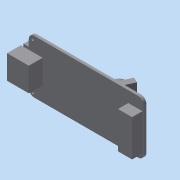
# Autodesk Inventor part: 00_ESP32_CAM
Saved by Autodesk Inventor 2019.4 (Build 234330000, 330)
## iProperties
Created: 2020-11-30
Part Number: 00_ESP32_CAM
Material: Generic
Document SubType Name: Modeling
Designer: diederichbenedict
Density: 1 g/cm^3
Appearance: Default
Author: diederichbenedict
Autodesk Inventor part; units mm, degrees
ref_plane "YZ Plane" through (0, 0, 0) normal (1, 0, 0) x (0, 1, 0)
ref_plane "XZ Plane" through (0, 0, 0) normal (0, 1, 0) x (-1, 0, 0)
ref_plane "XY Plane" through (0, 0, 0) normal (0, 0, 1) x (1, 0, 0)
sketch "Sketch1" plane through (0, 0, 0) normal (0, 0, 1) x (1, 0, 0)
  line L0 (19.65, -10.075) -> (-19.65, -10.075)
  line L1 (-21.65, -8.075) -> (-21.65, 8.075)
  line L2 (-19.65, 10.075) -> (19.65, 10.075)
  line L3 (21.65, 8.075) -> (21.65, -8.075)
  line L4 (21.65, -10.075) -> (-21.65, 10.075) construction
  line L5 (-21.65, -10.075) -> (21.65, 10.075) construction
  arc A0 (-19.65, 10.075) -> (-21.65, 8.075) centre (-19.65, 8.075) ccw
  arc A1 (21.65, 8.075) -> (19.65, 10.075) centre (19.65, 8.075) ccw
  arc A2 (19.65, -10.075) -> (21.65, -8.075) centre (19.65, -8.075) ccw
  arc A3 (-21.65, -8.075) -> (-19.65, -10.075) centre (-19.65, -8.075) ccw
  point P0 (0, 0)
  dimension "d0" = 43.3
  dimension "d1" = 20.15
  dimension "d2" = 2
  constraints: 12 end point, 8 point on circle, 8 point on line, 8 tangent, 4 centre point, 3 equal radius, 2 midpoint, 2 parallel, 1 horizontal, 1 perpendicular
  measures "d0" distance of L4.end L5.end
  measures "d1" distance of L5.start L4.end
  measures "d2" radius of A0
extrude "Extrusion1" add sketch "Sketch1" along normal blind 1
sketch "Sketch2" plane through (0, 0, 0) normal (0, 0, -1) x (-1, 0, 0)
  line L0 (19.65, 10.075) -> (-19.65, 10.075) projected
  arc A0 (-19.65, 10.075) -> (-21.65, 8.075) centre (-19.65, 8.075) ccw projected
  line L1 (-21.65, 8.075) -> (-21.65, -8.075) projected
  arc A1 (-21.65, -8.075) -> (-19.65, -10.075) centre (-19.65, -8.075) ccw projected
  line L2 (-19.65, -10.075) -> (19.65, -10.075) projected
  arc A2 (19.65, -10.075) -> (21.65, -8.075) centre (19.65, -8.075) ccw projected
  line L3 (21.65, -8.075) -> (21.65, 8.075) projected
  arc A3 (21.65, 8.075) -> (19.65, 10.075) centre (19.65, 8.075) ccw projected
  line L4 (17.25, -4.5) -> (24.65, -4.5)
  line L5 (24.65, -4.5) -> (24.65, 4.5)
  line L6 (24.65, 4.5) -> (17.25, 4.5)
  line L7 (17.25, 4.5) -> (17.25, -4.5)
  line L8 (17.25, -4.5) -> (24.65, 4.5) construction
  line L9 (24.65, -4.5) -> (17.25, 4.5) construction
  point P0 (0, 0)
  point P1 (20.95, 0)
  dimension "d5" = 7.4
  dimension "d6" = 9
  dimension "d7" = 3
  constraints: 12 end point, 2 midpoint, 2 parallel, 1 horizontal, 1 perpendicular
  measures "d5" distance of L6.end L5.end
  measures "d6" distance of L5.end L4.end
  measures "d7" distance between parallel lines of L3 L5
extrude "Extrusion2" add sketch "Sketch2" along normal blind 3 contours L6 L5 L4 L3 | L3 L4 L7 L6
sketch "Sketch3" plane through (0, 0, 1) normal (0, 0, 1) x (1, 0, 0)
  line L0 (-16.45, 4.5) -> (-24.65, 4.5)
  line L1 (-24.65, 4.5) -> (-24.65, -4.5)
  line L2 (-24.65, -4.5) -> (-16.45, -4.5)
  line L3 (-16.45, -4.5) -> (-16.45, 4.5)
  line L4 (-16.45, 4.5) -> (-24.65, -4.5) construction
  line L5 (-24.65, 4.5) -> (-16.45, -4.5) construction
  line L6 (-21.65, 8.075) -> (-21.65, -8.075) projected
  point P0 (0, 0)
  point P1 (-20.55, 0)
  dimension "d10" = 8.2
  dimension "d11" = 9
  dimension "d12" = 3
  constraints: 12 end point, 2 midpoint, 2 parallel, 1 horizontal, 1 perpendicular
  measures "d10" distance of L2.end L1.end
  measures "d11" distance of L1.end L0.end
  measures "d12" distance between parallel lines of L6 L1
extrude "Extrusion3" add sketch "Sketch3" along normal blind 5.2
sketch "Sketch4" plane through (0, 0, 1) normal (0, 0, 1) x (1, 0, 0)
  line L0 (21.1704, -7.925) -> (15.85, -7.925)
  line L1 (15.85, -7.925) -> (15.85, 5.875)
  line L2 (15.85, 5.875) -> (21.1704, 5.875)
  line L3 (21.1704, 5.875) -> (21.1704, -7.925)
  line L4 (-19.65, -10.075) -> (19.65, -10.075) projected
  line L5 (19.65, 10.075) -> (-19.65, 10.075) projected
  line L6 (21.65, -8.075) -> (21.65, 8.075) projected
  point P0 (0, 0)
  dimension "d15" = 2.15
  dimension "d16" = 4.2
  dimension "d17" = 5.8
  constraints: 8 end point, 2 parallel, 1 horizontal, 1 perpendicular
  measures "d15" distance between parallel lines of L0 L4
  measures "d16" distance between parallel lines of L2 L5
  measures "d17" distance between parallel lines of L6 L1
extrude "Extrusion4" add sketch "Sketch4" along normal blind 3.9
sketch "Sketch5" plane through (0, 0, 0) normal (0, 0, -1) x (-1, 0, 0)
  line L0 (17.25, 4.5) -> (21.65, 4.5) projected
  line L1 (21.65, 4.5) -> (21.65, 8.075) projected
  arc A0 (21.65, 8.075) -> (19.65, 10.075) centre (19.65, 8.075) ccw projected
  line L2 (19.65, 10.075) -> (-19.65, 10.075) projected
  arc A1 (-19.65, 10.075) -> (-21.65, 8.075) centre (-19.65, 8.075) ccw projected
  line L3 (-21.65, 8.075) -> (-21.65, -8.075) projected
  arc A2 (-21.65, -8.075) -> (-19.65, -10.075) centre (-19.65, -8.075) ccw projected
  line L4 (-19.65, -10.075) -> (19.65, -10.075) projected
  arc A3 (19.65, -10.075) -> (21.65, -8.075) centre (19.65, -8.075) ccw projected
  line L5 (21.65, -8.075) -> (21.65, -4.5) projected
  line L6 (21.65, -4.5) -> (17.25, -4.5) projected
  line L7 (17.25, -4.5) -> (17.25, 4.5) projected
  circle A4 centre (20.3112, 8.6013) radius 0.5
  circle A5 centre (20.3112, -8.8284) radius 0.5
  point P0 (0, 0)
  dimension "d20" = 1
  dimension "d21" = 1
  constraints: 2 centre point
  measures "d20" diameter of A4
  measures "d21" diameter of A5
extrude "Extrusion5" cut sketch "Sketch5" against normal blind 3.9 contours A4 | A5
sketch "Sketch6" plane through (0, 0, 0) normal (0, 1, 0) x (-1, 0, 0)
  line L0 (19.65, 0) -> (-19.65, 0) projected
  line L1 (-3.7519, 0) -> (-2.2949, -8.2628)
  line L2 (21.65, 0) -> (21.65, 1) projected
  line L3 (-3.6651, -0.4924) -> (-2.0849, -9.4542)
  line L4 (-2.0849, -9.4542) -> (0.1802, -9.0548)
  line L5 (0.1802, -9.0548) -> (-1.4, -0.093)
  line L6 (-1.4, -0.093) -> (-3.6651, -0.4924)
  line L7 (-3.6651, -0.4924) -> (0.1802, -9.0548) construction
  line L8 (-2.0849, -9.4542) -> (-1.4, -0.093) construction
  line L9 (-21.65, 0) -> (-21.65, 1) projected
  point P0 (0, 0)
  point P1 (-1.7424, -4.7736)
  dimension "deg_1" = 80
  dimension "d28" = 9.1
  dimension "d29" = 2.3
  dimension "d30" = 0.5
  dimension "d42" = 20.25
  constraints: 14 end point, 2 midpoint, 2 parallel, 2 point on line, 1 collinear, 1 perpendicular
  measures "deg_1" angle of L0 L1
  measures "d28" distance of L3.start L3.end
  measures "d29" distance of L4.end L3.end
  measures "d30" distance from line of L1.start L6
  measures "d42" distance from line of L9 L5.end
extrude "Extrusion6" add sketch "Sketch6" along normal mid plane 9.1
sketch "Sketch7" plane through (1.4, -4.55, -0.093) normal (-0.9848, 0, 0.1736) x (0.1736, 0, 0.9848)
  line L0 (0, 9.1) -> (0, 0) projected
  line L1 (-9.1, 9.1) -> (0, 9.1) projected
  line L2 (-9.1, 9.1) -> (-9.1, 0) projected
  line L3 (0, 0) -> (-9.1, 0) projected
  circle A0 centre (-4.55, 4.55) radius 4.15
  circle A1 centre (-4.55, 4.55) radius 3.5
  point P0 (-0.1515, 4.55)
  dimension "d33" = 8.3
  dimension "d34" = 7
  constraints: 2 centre point, 1 coincident
  measures "d33" diameter of A0
  measures "d34" diameter of A1
extrude "Extrusion7" add sketch "Sketch7" against normal blind 3.7 contours A0
sketch "Sketch8" plane through (0, 0, 0) normal (0, 0, -1) x (-1, 0, 0)
  line L0 (9.43, -8) -> (3.83, -8)
  line L1 (3.83, -8) -> (3.83, 8)
  line L2 (3.83, 8) -> (9.43, 8)
  line L3 (9.43, 8) -> (9.43, -8)
  line L4 (9.43, -8) -> (3.83, 8) construction
  line L5 (3.83, -8) -> (9.43, 8) construction
  line L6 (21.65, 4.5) -> (21.65, 8.075) projected
  point P0 (0, 0)
  point P1 (6.63, 0)
  dimension "d37" = 5.6
  dimension "d38" = 16
  dimension "d39" = 12.22
  constraints: 12 end point, 2 midpoint, 2 parallel, 1 horizontal, 1 perpendicular
  measures "d37" distance of L1.end L2.end
  measures "d38" distance of L0.end L1.end
  measures "d39" distance between parallel lines of L3 L6
extrude "Extrusion8" add sketch "Sketch8" along normal blind 2
body "Solid1"
